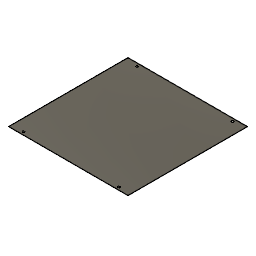
Sol 200x200mm (Autodesk Fusion 360 design; units mm, degrees)
part number: 2026-03-31-14-11-04-905
Autodesk Fusion 360 part; units mm, degrees
sketch "Esquisse1" plane through (0, 0, 0) normal (0, 0, 1) x (1, 0, 0)
  line L0 (0, 0) -> (200, 0)
  line L1 (200, 0) -> (200, 200)
  line L2 (200, 200) -> (0, 200)
  line L3 (0, 200) -> (0, 0)
  dimension "d18" = 200
  dimension "d19" = 200
  constraint horizontal L0
  constraint vertical L1
  constraint horizontal L2
  constraint vertical L3
  constraint coincident L0.start L3.end
  measures "d18" distance of L0 L2
  measures "d19" distance of L1 L3
extrude "Extrusion1" add sketch "Esquisse1" along normal blind 4
chamfer "Chanfrein1" distance 4 angle 45 1 faces at (66.6667, 133.3333, 0)
sketch "Esquisse2" plane through (0, 0, 4) normal (0, 0, 1) x (-1, 0, 0)
  circle A0 centre (-20, -195) radius 2
  circle A1 centre (-180, -195) radius 2
  circle A2 centre (-180, -5) radius 2
  circle A3 centre (-20, -5) radius 2
  line L0 (0, -200) -> (0, 0)
  line L1 (0, 0) -> (-200, 0)
  line L2 (-200, 0) -> (-200, -200)
  line L3 (-200, -200) -> (0, -200)
  line L4 (-20, -5) -> (-20, 0)
  line L5 (-180, -5) -> (-180, 0)
  line L6 (-20, -195) -> (-20, -200)
  line L7 (-180, -195) -> (-180, -200)
  line L8 (-20, -5) -> (0, -5)
  line L9 (-180, -5) -> (-200, -5)
  line L10 (-180, -195) -> (-200, -195)
  line L11 (-20, -195) -> (0, -195)
  dimension "d10" = 4
  dimension "d11" = 4
  dimension "d12" = 4
  dimension "d13" = 4
  dimension "d28" = 5
  dimension "d29" = 5
  dimension "d30" = 5
  dimension "d31" = 5
  dimension "d32" = 20
  dimension "d33" = 20
  dimension "d34" = 20
  dimension "d35" = 20
  constraint coincident A3.centre L4.start
  constraint coincident A2.centre L5.start
  constraint coincident A0.centre L6.start
  constraint coincident A1.centre L7.start
  constraint coincident L1 L4.end
  constraint perpendicular L1 L4
  constraint coincident L1 L5.end
  constraint perpendicular L1 L5
  constraint coincident L3 L6.end
  constraint perpendicular L3 L6
  constraint coincident L3 L7.end
  constraint perpendicular L3 L7
  constraint coincident L0 L8.end
  constraint perpendicular L0 L8
  constraint coincident L2 L9.end
  constraint perpendicular L2 L9
  constraint coincident L2 L10.end
  constraint perpendicular L2 L10
  constraint coincident L0 L11.end
  constraint perpendicular L0 L11
  measures "d10" diameter of A0
  measures "d11" diameter of A1
  measures "d12" diameter of A2
  measures "d13" diameter of A3
  measures "d28" distance of A3.centre L4.end
  measures "d29" distance of A2.centre L5.end
  measures "d30" distance of A0.centre L6.end
  measures "d31" distance of A1.centre L7.end
  measures "d32" distance of A3.centre L8.end
  measures "d33" distance of A2.centre L9.end
  measures "d34" distance of A0.centre L11.end
  measures "d35" distance of A1.centre L10.end
extrude "Extrusion2" cut sketch "Esquisse2" against normal blind 14 contours A0 L6 L11 | A0 L6 L11 | A3 L4 L8 | A3 L4 L8 | A1 L7 L10 | A1 L7 L10 | A2 L5 L9 | A2 L5 L9
thread "Filetage1" "ISO Metric profile 4.0 M4x0.7 M4x0.7 6H" major diameter 4.1095 minor diameter 3.332 pitch 0.7 angle 60 resizes the face on face at (18.3544, 196.1367, 1.4246)
thread "Filetage2" "ISO Metric profile 4.0 M4x0.7 M4x0.7 6H" major diameter 4.1095 minor diameter 3.332 pitch 0.7 angle 60 resizes the face on face at (21.6456, 3.8633, 1.4246)
thread "Filetage3" "ISO Metric profile 4.0 M4x0.7 M4x0.7 6H" major diameter 4.1095 minor diameter 3.332 pitch 0.7 angle 60 resizes the face on face at (181.6456, 3.8633, 1.4246)
thread "Filetage4" "ISO Metric profile 4.0 M4x0.7 M4x0.7 6H" major diameter 4.1095 minor diameter 3.332 pitch 0.7 angle 60 resizes the face on face at (178.3544, 196.1367, 1.4246)
move_face "DécalerLesFaces1" offset -0.05 1 faces at (21.5507, 5.6091, 2.6667)
move_face "DécalerLesFaces2" offset -0.05 1 faces at (181.5507, 5.6091, 2.6667)
move_face "DécalerLesFaces3" offset -0.05 1 faces at (181.5507, 194.3909, 2.6667)
move_face "DécalerLesFaces4" offset -0.05 1 faces at (21.5507, 194.3909, 2.6667)
